Autodesk Inventor part; units mm, degrees
(part 2 of 2)
  spline S37 degree 2 poles (-54.0998, 84.3858) (-54.462, 84.3858) (-55.2031, 84.2047) (-55.5406, 84.0647) knots 0 0 0 1 2 2 2
  spline S38 degree 2 poles (-55.5406, 84.0647) (-55.8288, 83.9495) (-56.364, 83.6201) (-56.5286, 83.5049) knots 0 0 0 1 2 2 2
  line L237 (-56.5286, 83.5049) -> (-56.6027, 83.5049)
  line L238 (-56.6027, 83.5049) -> (-56.6027, 84.9539)
  spline S39 degree 2 poles (-56.6027, 84.9539) (-56.1828, 85.1598) (-54.6761, 85.5632) (-54.001, 85.5632) knots 0 0 0 1 2 2 2
  spline S40 degree 2 poles (-54.001, 85.5632) (-52.5766, 85.5632) (-50.9711, 84.0565) (-50.9711, 82.7721) knots 0 0 0 1 2 2 2
  spline S41 degree 2 poles (-50.9711, 82.7721) (-50.9711, 82.1711) (-51.251, 81.1666) (-51.498, 80.7384) knots 0 0 0 1 2 2 2
  spline S42 degree 2 poles (-51.498, 80.7384) (-51.745, 80.2938) (-52.4613, 79.4211) (-52.8565, 79.0012) knots 0 0 0 1 2 2 2
  spline S43 degree 2 poles (-52.8565, 79.0012) (-53.4987, 78.3014) (-55.0713, 76.8029) (-55.5406, 76.3665) knots 0 0 0 1 2 2 2
  line L239 (-55.5406, 76.3665) -> (-50.5512, 76.3665)
  line L240 (-50.5512, 76.3665) -> (-50.5512, 75.1891)
  point P0 (-31.75, 68.8958)
  point P1 (-31.75, 20.0009)
  point P2 (-53.7479, 68.8958)
  point P3 (-9.7521, 20.0042)
  point P4 (-41.8348, 101.4209)
  point P5 (-31.75, 68.8958)
  point P6 (-31.75, 20.0009)
  point P7 (-53.7479, 68.8958)
  point P8 (-9.7521, 20.0042)
  point P9 (-1, 6.9835)
  dimension "d155" = 8.4153
  dimension "d157" = 0.508
  dimension "d158" = 4.5466
  dimension "d159" = 0.508
  dimension "d160" = 4.5466
  constraints: 408 end point, 25 parallel, 10 perpendicular, 7 horizontal, 1 midpoint, 9 other
  measures "d155" distance of L214.end L212.start
  measures "d157" distance between parallel lines of L7 L213
  measures "d158" distance from line of point (-1, 6.983) L212
  measures "d159" distance between parallel lines of L6 L208
  measures "d160" distance between parallel lines of L4 L211
extrude "Extrusion20" add sketch "Sketch17" along normal blind 0.4 contours L48 L49 L73 L71 L76 L69 L86 L79 L85 L67 L62 L68 L84 L80 L87 L77 L82 L60 L55 L61 L81 L78 L83 L70 L75 L72 L74 L50 | L88 L89 L113 L111 L116 L109 L126 L119 L125 L107 L102 L108 L124 L120 L127 L117 L122 L100 L95 L101 L121 L118 L123 L110 L115 L112 L114 L90 | L128 L129 L153 L151 L156 L149 L166 L159 L165 L147 L142 L148 L164 L160 L167 L157 L162 L140 L135 L141 L161 L158 L163 L150 L155 L152 L154 L130 | L168 L169 L193 L191 L196 L189 L206 L199 L205 L187 L182 L188 L204 L200 L207 L197 L202 L180 L175 L181 L201 L198 L203 L190 L195 L192 L194 L170 | L217 L218 S0 S1 S2 S3 S4 S5 L219 L220 S6 S7 S8 S9 S10 L221 L222 | L223 L224 S11 S12 S13 S14 S15 S16 L225 L226 S17 S18 S19 S20 S21 L227 L228 bodies 2
sketch "Sketch18" plane through (0, 0, -0.2) normal (0, 0, -1) x (-1, 0, 0)
  line L0 (0, 0) -> (-63.5, 0)
  line L1 (-63.5, 0) -> (-63.5, 88.9)
  line L2 (-63.5, 88.9) -> (0, 88.9)
  line L3 (0, 88.9) -> (0, 0)
  constraints: 8 end point, 2 parallel, 1 horizontal, 1 perpendicular
extrude "Extrusion21" add sketch "Sketch18" along normal blind 0.4 bodies 3
fillet "Fillet2" radius 3.175 8 edges at (63.5, 0, 0.2) (63.5, 88.9, 0.2) (0, 0, 0.2) (0, 88.9, 0.2) (63.5, 0, -0.3) (63.5, 88.9, -0.3) (0, 0, -0.3) (0, 88.9, -0.3)
extrude "Extrusion22" cut sketch "Sketch17" along normal blind 0.4 contours L48 L49 L73 L71 L76 L69 L86 L79 L85 L67 L62 L68 L84 L80 L87 L77 L82 L60 L55 L61 L81 L78 L83 L70 L75 L72 L74 L50 | L88 L89 L113 L111 L116 L109 L126 L119 L125 L107 L102 L108 L124 L120 L127 L117 L122 L100 L95 L101 L121 L118 L123 L110 L115 L112 L114 L90 | L128 L129 L153 L151 L156 L149 L166 L159 L165 L147 L142 L148 L164 L160 L167 L157 L162 L140 L135 L141 L161 L158 L163 L150 L155 L152 L154 L130 | L168 L169 L193 L191 L196 L189 L206 L199 L205 L187 L182 L188 L204 L200 L207 L197 L202 L180 L175 L181 L201 L198 L203 L190 L195 L192 L194 L170 | L217 L218 S0 S1 S2 S3 S4 S5 L219 L220 S6 S7 S8 S9 S10 L221 L222 | L223 L224 S11 S12 S13 S14 S15 S16 L225 L226 S17 S18 S19 S20 S21 L227 L228 bodies 3
